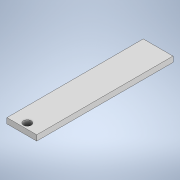
# Autodesk Inventor part: PX9200-24
Saved by Autodesk Inventor 2022.3 (Build 263350000, 350)
## iProperties
Created: 2022-07-15
Part Number: PX9200-24
Material: Generic
Document SubType Name: Modeling
Designer: luis_
Density: 1 g/cm^3
Appearance: Default
Author: luis_
Autodesk Inventor part; units mm, degrees
ref_plane "YZ Plane" through (0, 0, 0) normal (1, 0, 0) x (0, 1, 0)
ref_plane "XZ Plane" through (0, 0, 0) normal (0, 1, 0) x (-1, 0, 0)
ref_plane "XY Plane" through (0, 0, 0) normal (0, 0, 1) x (1, 0, 0)
sketch "Sketch1" plane through (0, 0, 0) normal (0, 1, 0) x (-1, 0, 0)
  line L0 (-9.5, 47.5) -> (9.5, 47.5)
  line L1 (9.5, 47.5) -> (9.5, -39.5)
  line L2 (6.5, -47.5) -> (-6.5, -47.5)
  line L3 (-9.5, -39.5) -> (-9.5, 47.5)
  line L4 (-9.5, 47.5) -> (9.5, -47.5) construction
  line L5 (9.5, 47.5) -> (-9.5, -47.5) construction
  line L6 (-6.5, -39.5) -> (6.5, -39.5)
  line L7 (6.5, -39.5) -> (6.5, -47.5)
  line L8 (6.5, -47.5) -> (-6.5, -47.5)
  line L9 (-6.5, -47.5) -> (-6.5, -39.5)
  line L10 (-6.5, -39.5) -> (6.5, -47.5) construction
  line L11 (6.5, -39.5) -> (-6.5, -47.5) construction
  line L12 (6.5, -39.5) -> (9.5, -39.5)
  line L13 (-6.5, -39.5) -> (-9.5, -39.5)
  point P0 (0, 0)
  point P1 (0, -43.5)
  dimension "d1" = 95
  constraints: 28 end point, 4 midpoint, 4 parallel, 3 perpendicular, 2 horizontal, 1 point on line
  measures "d1" distance of L0.end L4.end
extrude "Extrusion1" add sketch "Sketch1" along normal blind 3.5 contours L0 L1 L12 L6 L13 L3
sketch "Sketch2" plane through (0, 3.5, 0) normal (0, 1, 0) x (1, 0, 0)
  line L0 (-9.5, 39.5) -> (-9.5, -47.5) projected
  line L1 (-9.5, -46.5) -> (9.5, -46.5)
  line L2 (9.5, -47.5) -> (9.5, 39.5) projected
  line L3 (-9.5, -47.5) -> (9.5, -47.5) projected
  circle A0 centre (0, -44) radius 2.5
  point P0 (0, 0)
  point P1 (-9.5, 47.5)
  point P2 (9.5, 47.5)
  dimension "d5" = 1
  dimension "d6" = 5
  constraints: 2 end point, 2 point on line, 1 centre point, 1 tangent
  measures "d5" distance between parallel lines of L3 L1
  measures "d6" diameter of A0
extrude "Extrusion2" cut sketch "Sketch2" against normal blind 5 contours A0
body "Solid1"
